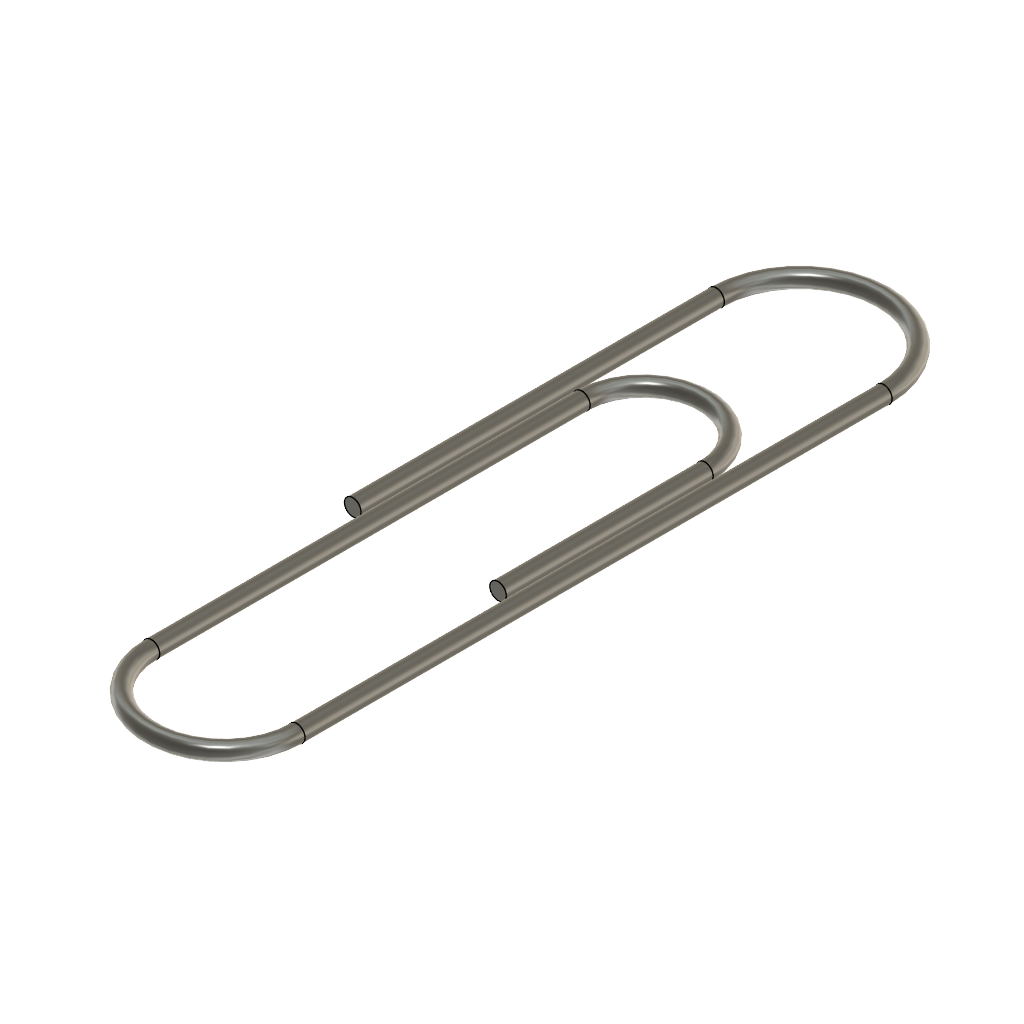
_Paper clip.78f07702-1bef-4d41-8cac-30635a14067d (Autodesk Fusion 360 design; units mm, degrees)
part number: 2026-09-21-15-04-57-308
Autodesk Fusion 360 part; units mm, degrees
sketch "Sketch1" plane through (0, 0, 0) normal (0, 0, 1) x (1, 0, 0)
sketch "Sketch2" plane through (0, 0, 0) normal (0, 0, 1) x (1, 0, 0)
  line L0 (0, 0) -> (0, 16.25)
  line L1 (0, 16.25) -> (7.5, 16.25) construction
  line L2 (7.5, 16.25) -> (7.5, -10)
  line L3 (7.5, -10) -> (1, -10) construction
  line L4 (1, -10) -> (1, 9.25)
  line L5 (1, 9.25) -> (6.5, 9.25) construction
  line L6 (6.5, 9.25) -> (6.5, 0)
  arc A0 (7.5, 16.25) -> (0, 16.25) centre (3.75, 16.25) ccw
  arc A1 (6.5, 9.25) -> (1, 9.25) centre (3.75, 9.25) ccw
  arc A2 (1, -10) -> (7.5, -10) centre (4.25, -10) ccw
  dimension "d1" = 16.25
  dimension "d2" = 26.25
  dimension "d3" = 19.25
  dimension "d4" = 5.5
  constraint coincident L0.start origin
  constraint vertical L0
  constraint perpendicular L0 L1
  constraint perpendicular L1 L2
  constraint perpendicular L2 L3
  constraint perpendicular L3 L4
  constraint perpendicular L4 L5
  constraint perpendicular L5 L6
  constraint tangent L0 A0
  constraint tangent L6 A1
  constraint tangent L4 A2
  measures "d1" distance of L0.start L0.end
  measures "d2" distance of L1.end L2.end
  measures "d3" distance of L3.end L4.end
  measures "d4" distance of L4.end L5.end
sketch "Sketch3" plane through (0, 0, 0) normal (0, 1, 0) x (1, 0, 0)
  circle A0 centre (0, 0) radius 0.375
  dimension "d5" = 0.75
  constraint coincident A0.centre origin
  measures "d5" diameter of A0
sweep "Sweep1" add profiles "Sketch3" path "Sketch2" along L0 A0 L2 A2 L4 A1 L6 section 1
